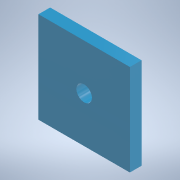
# Autodesk Inventor part: bold holder
Saved by Autodesk Inventor 2022 (Build 260153000, 153)
## iProperties
Created: 2021-05-28
Part Number: bold holder
Material: Silver
Document SubType Name: Modeling
Designer: benka
Density: 10.49 g/cm^3
Appearance: Sky Blue Dark
Author: benka
Autodesk Inventor part; units mm, degrees
ref_plane "YZ Plane" through (0, 0, 0) normal (1, 0, 0) x (0, 1, 0)
ref_plane "XZ Plane" through (0, 0, 0) normal (0, 1, 0) x (-1, 0, 0)
ref_plane "XY Plane" through (0, 0, 0) normal (0, 0, 1) x (1, 0, 0)
sketch "Sketch1" plane through (0, 0, 0) normal (0, 0, 1) x (1, 0, 0)
  circle A0 centre (0.002, 0.003) radius 2
  line L0 (-11.748, 11.753) -> (11.752, 11.753)
  line L1 (11.752, 11.753) -> (11.752, -11.747)
  line L2 (11.752, -11.747) -> (-11.748, -11.747)
  line L3 (-11.748, -11.747) -> (-11.748, 11.753)
  dimension "d5" = 4
  dimension "d8" = 23.5
  dimension "d9" = 23.5
  constraints: 8 end point, 2 parallel, 1 centre point, 1 horizontal, 1 perpendicular
  measures "d5" diameter of A0
  measures "d8" distance of L1.end L2.end
  measures "d9" distance of L0.end L1.end
extrude "Extrusion1" add sketch "Sketch1" along normal blind 3
body "Solid1"
